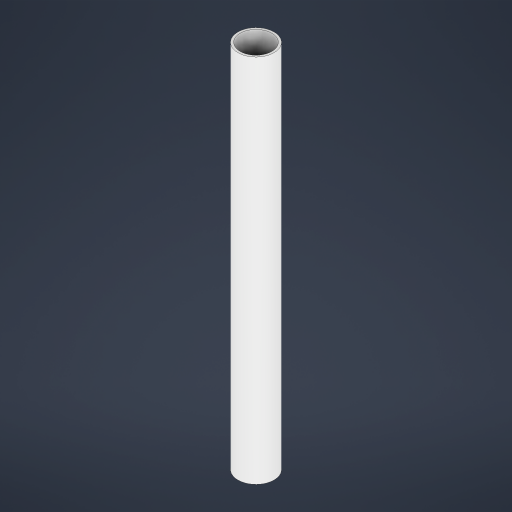
# Autodesk Inventor part: Shooter-pipes
Saved by Autodesk Inventor 2023 (Build 270158000, 158)
## iProperties
Created: 2022-04-13
Part Number: Shooter-pipes
Material: PVC-Piping
Document SubType Name: Modeling
Designer: timmy
Density: 1.4 g/cm^3
Appearance: Smooth - White
Author: timmy
Autodesk Inventor part; units mm, degrees
ref_plane "YZ Plane" through (0, 0, 0) normal (1, 0, 0) x (0, 1, 0)
ref_plane "XZ Plane" through (0, 0, 0) normal (0, 1, 0) x (-1, 0, 0)
ref_plane "XY Plane" through (0, 0, 0) normal (0, 0, 1) x (1, 0, 0)
sketch "Sketch1" plane through (0, 0, 0) normal (0, 1, 0) x (-1, 0, 0)
  circle A0 centre (0, 0) radius 44.45
  dimension "d0" = 88.9
  constraints: 1 centre point, 1 coincident
  measures "d0" diameter of A0
extrude "Extrusion1" add sketch "Sketch1" along normal blind 914.4
sketch "Sketch2" plane through (-27.4716, 0, -84.5489) normal (0, -1, 0) x (1, 0, 0)
  circle A0 centre (0, 0) radius 38.9636
  circle A1 centre (27.4716, 84.5489) radius 38.9636
  circle A2 centre (99.3932, 32.2948) radius 38.9636
  circle A3 centre (99.3932, 136.803) radius 38.9636
  circle A4 centre (0, 169.0978) radius 38.9636
  circle A5 centre (-61.4284, 84.5489) radius 38.9636
  dimension "d12" = 77.9272
  dimension "d16" = 360
  constraints: 6 centre point, 1 coincident, 11 other
  measures "d12" diameter of A0
extrude "Extrusion3" cut sketch "Sketch2" against normal through all contours A1
body "Solid1"
